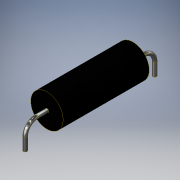
# Autodesk Inventor part: MT5-0R05F3_Power_Resistor
Saved by Autodesk Inventor 2016 (Build 200138000, 138)
## iProperties
Created: 2016-09-07
Part Number: MT5-0R05F3_Power_Resistor
Material: Generic
Document SubType Name: Modeling
Designer: jfixelle
Density: 1 g/cm^3
Appearance: Silver
Author: jfixelle
Autodesk Inventor part; units mm, degrees
ref_plane "YZ Plane" through (0, 0, 0) normal (1, 0, 0) x (0, 1, 0)
ref_plane "XZ Plane" through (0, 0, 0) normal (0, 1, 0) x (-1, 0, 0)
ref_plane "XY Plane" through (0, 0, 0) normal (0, 0, 1) x (1, 0, 0)
sketch "Sketch1" plane through (0, 0, 0) normal (0, 0, 1) x (1, 0, 0)
  circle A0 centre (0, 4.25) radius 4.25
  point P0 (0, 0)
  dimension "d0" = 8.5
  dimension "d1" = 4.25
  constraints: 1 centre point
  measures "d0" diameter of A0
  measures "d1" distance of point (0, 0) A0.centre
extrude "Extrusion1" add sketch "Sketch1" along normal mid plane 22.6
sketch "Sketch2" plane through (0, 4.25, 11.3) normal (0, 0, 1) x (1, 0, 0)
  circle A0 centre (0, 0) radius 0.5
  point P0 (0, -4.25)
  dimension "d4" = 1
  constraints: 1 centre point
  measures "d4" diameter of A0
sketch "Sketch3" plane through (0, 0, 0) normal (1, 0, 0) x (0, 1, 0)
  line L0 (8.5, 11.3) -> (0, 11.3) projected
  line L1 (4.25, 11.3) -> (4.25, 14)
  line L2 (1.25, 17) -> (-0.9549, 17)
  arc A0 (4.25, 14) -> (1.25, 17) centre (1.25, 14) ccw
  line L3 (-0.9549, 17) -> (-2, 17)
  point P0 (0, 0)
  dimension "d5" = 17
  dimension "d6" = 3
  dimension "d8" = 2
  constraints: 6 end point, 2 point on circle, 2 tangent, 1 centre point, 1 horizontal, 1 midpoint, 1 perpendicular, 1 vertical
  measures "d5" distance from line of point (0, 0) L2
  measures "d6" radius of A0
  measures "d8" horizontal distance of L3.end point (0, 0)
sweep "Sweep1" add profiles "Sketch2" path "Sketch3" path curves L1 A0 L2 L3
mirror "Mirror1" about plane through (0, 0, 0) normal (0, 0, 1) of "Sweep1"
body "Solid1"
